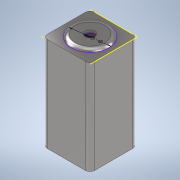
# Autodesk Inventor part: pneumatic_cylinder_ body
Saved by Autodesk Inventor 2022 (Build 260153000, 153)
## iProperties
Created: 2021-11-08
Part Number: pneumatic_cylinder_ body
Material: Stainless Steel
Document SubType Name: Modeling
Designer: kibandi
Density: 8 g/cm^3
Appearance: Semi-Polished
Author: kibandi
Autodesk Inventor part; units mm, degrees
ref_plane "YZ Plane" through (0, 0, 0) normal (1, 0, 0) x (0, 1, 0)
ref_plane "XZ Plane" through (0, 0, 0) normal (0, 1, 0) x (-1, 0, 0)
ref_plane "XY Plane" through (0, 0, 0) normal (0, 0, 1) x (1, 0, 0)
sketch "Sketch1" plane through (0, 0, 0) normal (0, 1, 0) x (-1, 0, 0)
  line L0 (0, 0) -> (-100, 0)
  line L1 (-100, 0) -> (-100, -100)
  line L2 (-100, -100) -> (0, -100)
  line L3 (0, -100) -> (0, 0)
  dimension "d0" = 100
  dimension "d1" = 100
  constraints: 8 end point, 2 parallel, 1 horizontal, 1 perpendicular
  measures "d0" distance of L2.end L1.end
  measures "d1" distance of L1.end L0.end
extrude "Extrusion1" add sketch "Sketch1" along normal blind 200
sketch "Sketch2" plane through (0, 200, 0) normal (0, 1, 0) x (1, 0, 0)
  line L0 (100, 0) -> (100, 100) projected
  line L1 (100, 100) -> (0, 100) projected
  circle A0 centre (50, 50) radius 10
  circle A1 centre (50, 50) radius 40
  point P0 (0, 0)
  dimension "d4" = 20
  dimension "d5" = 80
  constraints: 2 centre point, 1 coincident
  measures "d4" diameter of A0
  measures "d5" diameter of A1
extrude "Extrusion2" cut sketch "Sketch2" against normal blind 175 contours A0
extrude "Extrusion3" add sketch "Sketch2" along normal blind 5
fillet "Fillet1" radius 10 1 edges at (10, 205, -50)
fillet "Fillet2" radius 10 4 edges at (100, 100, 0) (0, 100, 0) (0, 100, -100) (100, 100, -100)
body "Solid1"
